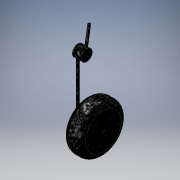
# Autodesk Inventor part: Nose Gear Rod and Wheel
Saved by Autodesk Inventor 2018 (Build 220112000, 112)
## iProperties
Created: 2018-08-04
Part Number: Nose Gear Rod and Wheel
Material: Generic
Document SubType Name: Modeling
Designer: Michael Gunderman
Density: 0.739747 g/cm^3
Appearance: Default
Mass: 88 g
Surface Area: 166.864 cm^2
Volume: 118.96 cm^3
Author: Michael Gunderman
Autodesk Inventor part; units mm, degrees
ref_plane "Work Plane1" through (0, 91, 0) normal (0.9999, 0.0142, 0) x (-0.0142, 0.9999, 0)
sketch "Sketch1" plane through (0, 91, 0) normal (0.9999, 0.0142, 0) x (-0.0142, 0.9999, 0)
  circle A0 centre (0, 0) radius 8.95
  point P0 (-90.9908, 0)
  dimension "d3" = 17.9
  constraints: 1 centre point
  measures "d3" diameter of A0
extrude "Extrusion1" add sketch "Sketch1" along normal blind 14
ref_plane "Work Plane2" through (40.3, 0, 0) normal (1, 0, 0) x (0, 1, 0)
sketch "Sketch2" plane through (40.3, 0, 0) normal (1, 0, 0) x (0, 1, 0)
  circle A0 centre (0, 0) radius 2
  dimension "d6" = 4
  constraints: 1 centre point, 1 coincident
  measures "d6" diameter of A0
ref_plane "Work Plane3" through (11.5062, 129.8959, -6.5569) normal (-0.0002, -0.986, 0.1669) x (1, -0.0002, 0)
sketch "Sketch3" plane through (11.5062, 129.8959, -6.5569) normal (-0.0002, -0.986, 0.1669) x (1, -0.0002, 0)
  circle A0 centre (0, 0) radius 2
  point P0 (-11.4815, -15.2165)
  dimension "d7" = 4
  constraints: 1 centre point
  measures "d7" diameter of A0
sketch3d "3D Sketch1"
  line L0 (11.5062, 129.8959, -6.5569) -> (11.4988, 91.1633, 0)
  dimension "d0" = 40.3
  dimension "d1" = 91
  dimension "d2" = 11.5
sweep "Sweep1" add profiles "Sketch3" path "3D Sketch1"
sketch3d "3D Sketch1 for Sweep2"
  line L0 (40.3, 0, 0) -> (0, 0, 0)
  line L1 (0, 0, 0) -> (0, 91, 0)
  dimension "d0" = 40.3
  dimension "d1" = 91
  dimension "d2" = 11.5
sweep "Sweep2" add profiles "Sketch2" path "3D Sketch1 for Sweep2"
sketch "Sketch4" plane through (40.3, 0, 0) normal (1, 0, 0) x (0, 1, 0)
  circle A0 centre (0, 0) radius 38.1
  dimension "d12" = 76.2
  constraints: 1 centre point, 1 coincident
  measures "d12" diameter of A0
extrude "Extrusion2" add sketch "Sketch4" against normal blind 27 separate body
fillet "Fillet1" radius 10 2 edges at (40.3, -38.1, 0) (13.3, -38.1, 0)
body "Solid1"
body "Solid2"
